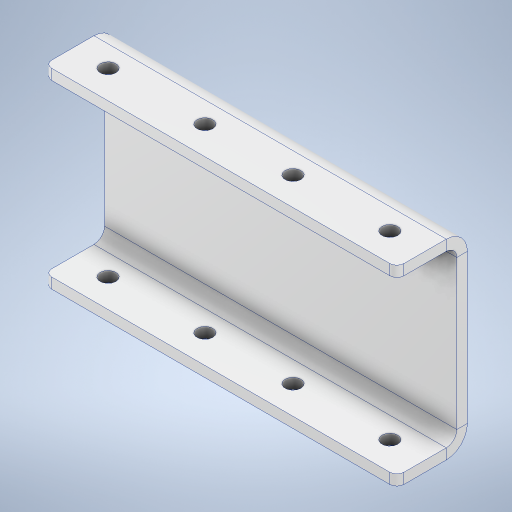
# Autodesk Inventor part: Seitenteil_03
Saved by Autodesk Inventor 2024 (Build 280153000, 153)
## iProperties
Created: 2024-03-25
Part Number: Seitenteil_03
Material: Aluminium 6061
Document SubType Name: Sheet Metal
Designer: month
Density: 2.7 g/cm^3
Sheet Metal Rule: Standard
Appearance: Aluminium - flach
Flat Pattern Width: 8.38717 cm
Flat Pattern Length: 10 cm
Flat Pattern Area: 83.8717 cm^2
Sheet Metal Width: 83,872 mm
Sheet Metal Length: 100,000 mm
Sheet Metal Area: 8387,168 mm^2
Author: month
Autodesk Inventor part; units mm, degrees
ref_plane "YZ Plane" through (0, 0, 0) normal (1, 0, 0) x (0, 1, 0)
ref_plane "XZ Plane" through (0, 0, 0) normal (0, 1, 0) x (-1, 0, 0)
ref_plane "XY Plane" through (0, 0, 0) normal (0, 0, 1) x (1, 0, 0)
sketch "Skizze1" plane through (0, 0, 0) normal (0, 1, 0) x (-1, 0, 0)
  line L0 (100, 0) -> (0, 0)
  line L1 (0, 0) -> (0, -42.3)
  line L2 (0, -42.3) -> (100, -42.3)
  line L3 (100, -42.3) -> (100, 0)
  dimension "d0" = 100
  dimension "d1" = 42.3
  constraints: 8 end point, 2 parallel, 1 coincident, 1 horizontal, 1 perpendicular
  measures "d0" distance of L1.end L2.end
  measures "d1" distance of L0.end L1.end
extrude "Extrusion1" add sketch "Skizze1" along normal blind 3
sketch "Skizze2" plane through (0, -3, -45.3) normal (0, 0, -1) x (-1, 0, 0)
  line L0 (100, 0) -> (0, 0)
  line L1 (0, 0) -> (0, -14)
  line L2 (0, -14) -> (100, -14)
  line L3 (100, -14) -> (100, 0)
  constraints: 6 end point, 1 horizontal, 1 perpendicular, 1 vertical
edge flange "Lasche1" height 20 angle 90 thickness 3 bend radius 3 thickness toward (0, 0, -1) relief tear relief width 3 relief depth 1.5 edges at (-50, 0, -42.3) wall of the first edge with corners at (-100, -3, -45.3) (0, -3, -45.3) (0, -17, -45.3) (-100, -17, -45.3)
bend "Biegung1"
corner "Ecke1"
sketch "Skizze3" plane through (-100, -3, 3) normal (0, 0, 1) x (1, 0, 0)
  line L0 (100, 0) -> (0, 0)
  line L1 (0, 0) -> (0, -14)
  line L2 (0, -14) -> (100, -14)
  line L3 (100, -14) -> (100, 0)
  constraints: 6 end point, 1 horizontal, 1 perpendicular, 1 vertical
edge flange "Lasche2" height 20 angle 90 thickness 3 bend radius 3 thickness toward (0, 0, 1) relief tear relief width 3 relief depth 1.5 edges at (-50, 0, 0) wall of the first edge with corners at (0, -3, 3) (-100, -3, 3) (-100, -17, 3) (0, -17, 3)
bend "Biegung2"
corner "Ecke2"
fillet "Rundung1" radius 2 4 edges at (-100, -17, -46.8) (-100, -17, 4.5) (0, -17, 4.5) (0, -17, -46.8)
sketch "Skizze4" plane through (-100, -3, 6) normal (0, 0, 1) x (1, 0, 0)
  line L0 (0, 0) -> (0, -12) projected
  line L1 (0, -6) -> (100, -6)
  line L2 (100, -12) -> (100, 0) projected
  line L3 (2, -14) -> (98, -14) projected
  line L4 (50, -14) -> (50, 0)
  circle A0 centre (90, -6) radius 2.25
  circle A1 centre (62.5, -6) radius 2.25
  circle A2 centre (37.5, -6) radius 2.25
  circle A3 centre (10, -6) radius 2.25
  point P0 (100, 3)
  dimension "d26" = 4.5
  dimension "d27" = 4.5
  dimension "d28" = 4.5
  dimension "d29" = 4.5
  dimension "d30" = 25
  dimension "d31" = 80
  constraints: 4 centre point, 4 end point, 4 point on line, 3 midpoint, 2 symmetric about line, 1 vertical
  measures "d26" diameter of A0
  measures "d27" diameter of A1
  measures "d28" diameter of A2
  measures "d29" diameter of A3
  measures "d30" distance of A2.centre A1.centre
  measures "d31" distance of A3.centre A0.centre
extrude "Extrusion2" cut sketch "Skizze4" against normal blind 100
equation "\"d4\" = Stärke"
equation "\"d5\" = BreiteBiegungsfreistellung"
equation "\"d6\" = TiefeBiegungsfreistellung"
equation "\"d7\" = MinimalRest"
equation "\"d8\" = Übergangsradius"
equation "\"d11\" = Biegeradius"
equation "\"d12\" = GrößeEckenfreistellung"
equation "\"d13\" = Abstandsgröße"
equation "\"d14\" = JacobiRadiusGröße"
equation "\"d15\" = BreiteBiegungsfreistellung"
equation "\"d16\" = TiefeBiegungsfreistellung"
equation "\"d17\" = MinimalRest"
equation "\"d18\" = Übergangsradius"
equation "\"d21\" = Biegeradius"
equation "\"d22\" = GrößeEckenfreistellung"
equation "\"d23\" = Abstandsgröße"
equation "\"d24\" = JacobiRadiusGröße"
equation "\"Biegeradius\" = Stärke"
equation "\"BreiteBiegungsfreistellung\" = Stärke"
equation "\"TiefeBiegungsfreistellung\" = 0.5 * Stärke"
equation "\"GrößeEckenfreistellung\" = 4 * Stärke"
equation "\"MinimalRest\" = 2 * Stärke"
equation "\"Übergangsradius\" = Biegeradius"
equation "\"JacobiRadiusGröße\" = Biegeradius"
equation "\"Abstandsgröße\" = Stärke"
equation "\"Stärke\" = 3"
